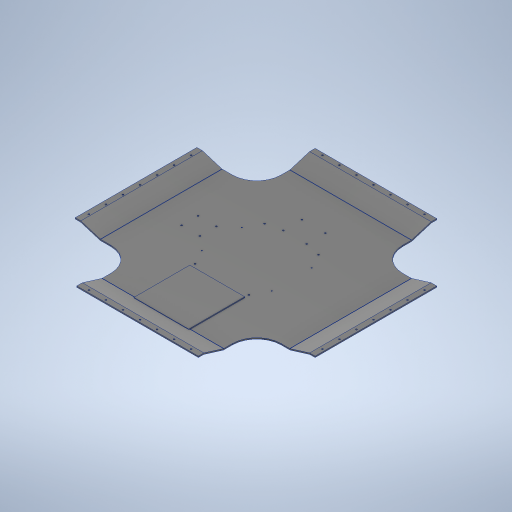
# Autodesk Inventor part: Swerve-Electronic-Plate
Saved by Autodesk Inventor 2024.2 (Build 282272000, 272)
## iProperties
Created: 2024-01-04
Part Number: Swerve-Electronic-Plate
Material: Aluminum 6061
Document SubType Name: Modeling
Designer: rohan
Density: 2.7 g/cm^3
Appearance: Aluminum - Flat
Author: rohan
Autodesk Inventor part; units mm, degrees
ref_plane "YZ Plane" through (0, 0, 0) normal (1, 0, 0) x (0, 1, 0)
ref_plane "XZ Plane" through (0, 0, 0) normal (0, 1, 0) x (-1, 0, 0)
ref_plane "XY Plane" through (0, 0, 0) normal (0, 0, 1) x (1, 0, 0)
sketch "Sketch6" plane through (0, 0, 0) normal (0, 1, 0) x (-1, 0, 0)
  line L0 (311.15, 311.15) -> (-311.15, 311.15)
  line L1 (-311.15, 311.15) -> (-311.15, -311.15)
  line L2 (-311.15, -311.15) -> (311.15, -311.15)
  line L3 (311.15, -311.15) -> (311.15, 311.15)
  line L4 (311.15, 311.15) -> (-311.15, -311.15) construction
  line L5 (-311.15, 311.15) -> (311.15, -311.15) construction
  point P0 (0, 0)
  dimension "d60" = 622.3
  dimension "d61" = 622.3
  constraints: 12 end point, 2 midpoint, 2 parallel, 1 horizontal, 1 perpendicular
  measures "d60" distance of L2.end L1.end
  measures "d61" distance of L1.end L0.end
extrude "Extrusion5" add sketch "Sketch6" along normal blind 3.175
sketch "Sketch7" plane through (0, 3.175, 0) normal (0, 1, 0) x (1, 0, 0)
  line L0 (311.15, -311.15) -> (311.15, 311.15) projected
  line L1 (311.15, 311.15) -> (-311.15, 311.15) projected
  line L2 (-311.15, 311.15) -> (-311.15, -311.15) projected
  line L3 (-311.15, -311.15) -> (311.15, -311.15) projected
  line L4 (-298.45, -298.45) -> (-298.45, 298.45)
  line L5 (-298.45, 298.45) -> (298.45, 298.45)
  line L6 (298.45, 298.45) -> (298.45, -298.45)
  line L7 (298.45, -298.45) -> (-298.45, -298.45)
  line L8 (0, -298.45) -> (0, -311.15)
  circle A0 centre (0, -304.8) radius 1.9939
  circle A1 centre (44.45, -304.8) radius 1.9939
  circle A2 centre (88.9, -304.8) radius 1.9939
  circle A3 centre (133.35, -304.8) radius 1.9939
  circle A4 centre (-44.45, -304.8) radius 1.9939
  circle A5 centre (0, -304.8) radius 1.9939
  circle A6 centre (44.45, -304.8) radius 1.9939
  circle A7 centre (88.9, -304.8) radius 1.9939
  circle A8 centre (-88.9, -304.8) radius 1.9939
  circle A9 centre (-44.45, -304.8) radius 1.9939
  circle A10 centre (0, -304.8) radius 1.9939
  circle A11 centre (44.45, -304.8) radius 1.9939
  circle A12 centre (-133.35, -304.8) radius 1.9939
  circle A13 centre (-88.9, -304.8) radius 1.9939
  circle A14 centre (-44.45, -304.8) radius 1.9939
  circle A15 centre (0, -304.8) radius 1.9939
  line L9 (-413.2249, 0) -> (395.3055, 0)
  line L10 (298.45, 298.45) -> (-298.45, 298.45)
  line L11 (0, 298.45) -> (0, 311.15)
  circle A16 centre (0, 304.8) radius 1.9939
  circle A17 centre (44.45, 304.8) radius 1.9939
  circle A18 centre (88.9, 304.8) radius 1.9939
  circle A19 centre (133.35, 304.8) radius 1.9939
  circle A20 centre (-44.45, 304.8) radius 1.9939
  circle A21 centre (0, 304.8) radius 1.9939
  circle A22 centre (44.45, 304.8) radius 1.9939
  circle A23 centre (88.9, 304.8) radius 1.9939
  circle A24 centre (-88.9, 304.8) radius 1.9939
  circle A25 centre (-44.45, 304.8) radius 1.9939
  circle A26 centre (0, 304.8) radius 1.9939
  circle A27 centre (44.45, 304.8) radius 1.9939
  circle A28 centre (-133.35, 304.8) radius 1.9939
  circle A29 centre (-88.9, 304.8) radius 1.9939
  circle A30 centre (-44.45, 304.8) radius 1.9939
  circle A31 centre (0, 304.8) radius 1.9939
  line L12 (-311.15, 0) -> (-298.45, 0)
  circle A32 centre (-304.8, 0) radius 1.9939
  circle A33 centre (-304.8, -44.45) radius 1.9939
  circle A34 centre (-304.8, -88.9) radius 1.9939
  circle A35 centre (-304.8, -133.35) radius 1.9939
  circle A36 centre (-304.8, 44.45) radius 1.9939
  circle A37 centre (-304.8, 0) radius 1.9939
  circle A38 centre (-304.8, -44.45) radius 1.9939
  circle A39 centre (-304.8, -88.9) radius 1.9939
  circle A40 centre (-304.8, 88.9) radius 1.9939
  circle A41 centre (-304.8, 44.45) radius 1.9939
  circle A42 centre (-304.8, 0) radius 1.9939
  circle A43 centre (-304.8, -44.45) radius 1.9939
  circle A44 centre (-304.8, 133.35) radius 1.9939
  circle A45 centre (-304.8, 88.9) radius 1.9939
  circle A46 centre (-304.8, 44.45) radius 1.9939
  circle A47 centre (-304.8, 0) radius 1.9939
  line L13 (0, 372.2506) -> (0, -355.6631)
  circle A48 centre (304.8, 0) radius 1.9939
  circle A49 centre (304.8, -44.45) radius 1.9939
  circle A50 centre (304.8, -88.9) radius 1.9939
  circle A51 centre (304.8, -133.35) radius 1.9939
  circle A52 centre (304.8, 44.45) radius 1.9939
  circle A53 centre (304.8, 0) radius 1.9939
  circle A54 centre (304.8, -44.45) radius 1.9939
  circle A55 centre (304.8, -88.9) radius 1.9939
  circle A56 centre (304.8, 88.9) radius 1.9939
  circle A57 centre (304.8, 44.45) radius 1.9939
  circle A58 centre (304.8, 0) radius 1.9939
  circle A59 centre (304.8, -44.45) radius 1.9939
  circle A60 centre (304.8, 133.35) radius 1.9939
  circle A61 centre (304.8, 88.9) radius 1.9939
  circle A62 centre (304.8, 44.45) radius 1.9939
  circle A63 centre (304.8, 0) radius 1.9939
  point P0 (0, 0)
  dimension "d64" = 12.7
  dimension "d65" = 3.9878
  dimension "d68" = 44.45
  dimension "d71" = 44.45
  dimension "d74" = 3.9878
  dimension "d77" = 44.45
  dimension "d80" = 44.45
  constraints: 64 centre point, 34 symmetric about line, 20 end point, 6 midpoint, 3 horizontal, 2 point on line, 2 vertical, 1 perpendicular, 95 other
  measures "d64" distance between parallel lines of L2 L4
  measures "d65" diameter of A0
  measures "d68" distance of A0.centre A1.centre
  measures "d71" distance of A0.centre A4.centre
  measures "d74" diameter of A32
  measures "d77" distance of A32.centre A33.centre
  measures "d80" distance of A32.centre A36.centre
extrude "Extrusion6" cut sketch "Sketch7" against normal blind 3.175 contours A48 L9 | L9 A48 | A0 L8 | L8 A0 | A16 L11 | L11 A16 | A32 L9 | L9 A32 | A1 | A2 | A3 | A4 | A8 | A12 | A17 | A18 | A19 | A20 | A24 | A28 | A33 | A34 | A35 | A36 | A40 | A44 | A49 | A50 | A51 | A52 | A56 | A60
sketch "Sketch8" plane through (0, 3.175, 0) normal (0, 1, 0) x (1, 0, 0)
  line L0 (-311.15, 311.15) -> (-311.15, -311.15) projected
  circle A0 centre (-304.8, 88.9) radius 1.9939 projected
  circle A1 centre (-304.8, -133.35) radius 1.9939 projected
  circle A2 centre (0, -304.8) radius 1.9939 projected
  circle A3 centre (304.8, -133.35) radius 1.9939 projected
  circle A4 centre (304.8, 44.45) radius 1.9939 projected
  circle A5 centre (88.9, 304.8) radius 1.9939 projected
  circle A6 centre (-88.9, 304.8) radius 1.9939 projected
  circle A7 centre (-44.45, 304.8) radius 1.9939 projected
  circle A8 centre (133.35, 304.8) radius 1.9939 projected
  circle A9 centre (304.8, 0) radius 1.9939 projected
  circle A10 centre (133.35, -304.8) radius 1.9939 projected
  circle A11 centre (-44.45, -304.8) radius 1.9939 projected
  circle A12 centre (-304.8, -88.9) radius 1.9939 projected
  circle A13 centre (-304.8, 133.35) radius 1.9939 projected
  circle A14 centre (-304.8, 44.45) radius 1.9939 projected
  circle A15 centre (-133.35, -304.8) radius 1.9939 projected
  circle A16 centre (44.45, -304.8) radius 1.9939 projected
  circle A17 centre (304.8, -88.9) radius 1.9939 projected
  circle A18 centre (304.8, 88.9) radius 1.9939 projected
  circle A19 centre (44.45, 304.8) radius 1.9939 projected
  circle A20 centre (-133.35, 304.8) radius 1.9939 projected
  circle A21 centre (0, 304.8) radius 1.9939 projected
  circle A22 centre (304.8, 133.35) radius 1.9939 projected
  circle A23 centre (304.8, -44.45) radius 1.9939 projected
  circle A24 centre (88.9, -304.8) radius 1.9939 projected
  circle A25 centre (-88.9, -304.8) radius 1.9939 projected
  circle A26 centre (-304.8, -44.45) radius 1.9939 projected
  circle A27 centre (-304.8, 0) radius 1.9939 projected
  line L1 (311.15, -311.15) -> (311.15, 311.15) projected
  line L2 (311.15, 311.15) -> (-311.15, 311.15) projected
  line L3 (-311.15, 311.15) -> (-311.15, -311.15) projected
  line L4 (-311.15, -311.15) -> (311.15, -311.15) projected
  line L5 (311.15, 311.15) -> (-311.15, 311.15) projected
  line L6 (-158.75, 311.15) -> (-158.75, 222.25)
  line L7 (-222.25, 158.75) -> (-311.15, 158.75)
  line L8 (-311.15, -158.75) -> (-222.25, -158.75)
  line L9 (-158.75, -222.25) -> (-158.75, -311.15)
  line L10 (158.75, 311.15) -> (158.75, 222.25)
  line L11 (222.25, 158.75) -> (311.15, 158.75)
  line L12 (158.75, -311.15) -> (158.75, -222.25)
  line L13 (222.25, -158.75) -> (311.15, -158.75)
  arc A28 (-222.25, 158.75) -> (-158.75, 222.25) centre (-222.25, 222.25) ccw
  arc A29 (158.75, 222.25) -> (222.25, 158.75) centre (222.25, 222.25) ccw
  arc A30 (222.25, -158.75) -> (158.75, -222.25) centre (222.25, -222.25) ccw
  arc A31 (-158.75, -222.25) -> (-222.25, -158.75) centre (-222.25, -222.25) ccw
  point P0 (0, 0)
  point P1 (-311.15, 0)
  point P2 (0, 311.15)
  point P3 (-158.75, 158.75)
  point P4 (-158.75, -158.75)
  point P5 (158.75, 158.75)
  point P6 (0, -311.15)
  point P7 (158.75, -158.75)
  dimension "d93" = 63.5
  constraints: 18 point on line, 16 end point, 8 point on circle, 8 tangent, 4 centre point, 3 equal radius, 3 midpoint, 2 parallel, 2 perpendicular, 2 vertical
  measures "d93" radius of A28
extrude "Extrusion8" cut sketch "Sketch8" against normal blind 61.9125 contours L2 L6 A28 L7 L0 | L8 A31 L9 L4 L0 | L2 L1 L11 A29 L10 | L12 A30 L13 L1 L4
sketch "Sketch17" plane through (158.75, 3.175, 311.15) normal (1, 0, 0) x (0, 0, -1)
  line L0 (88.9, -3.175) -> (0, -3.175) projected
  line L1 (88.9, -3.175) -> (0, -3.175) projected
  line L2 (88.9, 0) -> (88.9, -3.175) projected
  line L3 (0, 0) -> (88.9, 0) projected
  line L4 (0, -3.175) -> (0, 0) projected
  line L5 (622.3, -3.175) -> (533.4, -3.175) projected
  line L6 (622.3, 0) -> (622.3, -3.175) projected
  line L7 (533.4, 0) -> (622.3, 0) projected
  line L8 (533.4, 0) -> (533.4, -3.175) projected
  line L9 (4.3561, 0) -> (8.3439, 0) projected
  line L10 (0, 12.7) -> (13.97, 12.7)
  line L11 (13.97, 12.7) -> (55.1332, 0)
  line L12 (152.4, 0) -> (469.9, 0) projected
  line L13 (311.15, 0) -> (311.15, 175.4287)
  line L14 (622.3, 12.7) -> (608.33, 12.7)
  line L15 (608.33, 12.7) -> (567.1668, 0)
  line L16 (56.0693, 3.0339) -> (14.4487, 15.875)
  line L17 (14.4487, 15.875) -> (0, 15.875)
  line L18 (51.3204, 4.499) -> (65.9027, 0)
  line L19 (0, 12.7) -> (0, 15.875)
  line L20 (622.3, 12.7) -> (608.33, 12.7)
  line L21 (608.33, 12.7) -> (567.1668, 0)
  line L22 (566.2307, 3.0339) -> (607.8513, 15.875)
  line L23 (607.8513, 15.875) -> (622.3, 15.875)
  line L24 (570.9796, 4.499) -> (556.3973, 0)
  line L25 (622.3, 12.7) -> (622.3, 15.875)
  point P0 (311.15, -3.175)
  point P1 (567.1668, 0)
  point P2 (56.0693, 3.0339)
  dimension "d150" = 13.97
  dimension "d151" = 13.97
  dimension "d152" = 3.175
  dimension "d153" = 12.7
  constraints: 30 end point, 8 symmetric about line, 6 point on line, 1 midpoint, 1 perpendicular, 1 vertical
  measures "d150" distance of L10.start L10.end
  measures "d151" distance of L14.start L15.start
  measures "d152" distance between parallel lines of L11 L16
  measures "d153" distance of L3.start L10.start
extrude "Extrusion17" add sketch "Sketch17" against normal up to surface (317.5 mm away) contours L3 L11 L10 L19 L17 L16 L18 | L7 L24 L22 L23 L25 L14 L15
sketch "Sketch18" plane through (311.15, 3.175, -158.75) normal (0, 0, -1) x (-1, 0, 0)
  line L0 (88.9, -3.175) -> (0, -3.175) projected
  line L1 (88.9, 0) -> (88.9, -3.175) projected
  line L2 (0, 0) -> (88.9, 0) projected
  line L3 (0, -3.175) -> (0, 0) projected
  line L4 (622.3, -3.175) -> (533.4, -3.175) projected
  line L5 (622.3, 0) -> (622.3, -3.175) projected
  line L6 (533.4, 0) -> (622.3, 0) projected
  line L7 (533.4, 0) -> (533.4, -3.175) projected
  line L8 (152.4, 0) -> (469.9, 0) projected
  line L9 (309.1561, 0) -> (313.1439, 0) projected
  line L10 (313.1439, 0) -> (313.1439, 161.3413)
  line L11 (0, 12.7) -> (13.97, 12.7)
  line L12 (13.97, 12.7) -> (55.1338, 0)
  line L13 (88.9, 0) -> (0, 0) projected
  line L14 (56.0698, 3.0339) -> (14.4486, 15.875)
  line L15 (14.4486, 15.875) -> (0, 15.875)
  line L16 (0, 12.7) -> (0, 15.875)
  line L17 (54.6659, 3.467) -> (65.9034, 0)
  line L18 (626.2878, 12.7) -> (612.3178, 12.7)
  line L19 (612.3178, 12.7) -> (571.154, 0)
  line L20 (570.218, 3.0339) -> (611.8392, 15.875)
  line L21 (611.8392, 15.875) -> (626.2878, 15.875)
  line L22 (626.2878, 12.7) -> (626.2878, 15.875)
  line L23 (571.6219, 3.467) -> (560.3844, 0)
  point P0 (311.15, -3.175)
  point P1 (571.154, 0)
  point P2 (55.1338, 0)
  point P3 (56.0698, 3.0339)
  dimension "d157" = 13.97
  dimension "d158" = 43.0784
  dimension "d159" = 3.175
  dimension "d160" = 12.7
  constraints: 26 end point, 8 symmetric about line, 6 point on line, 1 perpendicular, 1 vertical
  measures "d157" distance of L11.start L11.end
  measures "d158" distance of L11.end L12.end
  measures "d159" distance between parallel lines of L12 L14
  measures "d160" distance of L11.start L2.start
extrude "Extrusion18" add sketch "Sketch18" against normal up to surface (317.5 mm away) contours L2 L12 L11 L16 L15 L14 L17 | L6 L23 L20 L21 L22 L18 L19
sketch "Sketch19" plane through (296.7014, 19.05, -158.75) normal (0, 1, 0) x (1, 0, 0)
  line L0 (-455.4514, -469.9) -> (-455.4514, -455.4513) projected
  line L1 (-137.9514, -469.9) -> (-455.4514, -469.9) projected
  line L2 (-137.9514, -455.4513) -> (-137.9514, -469.9) projected
  line L3 (-137.9514, -455.4513) -> (-455.4514, -455.4513) projected
  line L4 (14.4486, -317.5) -> (0, -317.5) projected
  line L5 (14.4486, 0) -> (14.4486, -317.5) projected
  line L6 (0, 0) -> (14.4486, 0) projected
  line L7 (0, 0) -> (0, -317.5) projected
  line L8 (-597.3905, -317.5) -> (-611.8392, -317.5) projected
  line L9 (-597.3905, 0) -> (-597.3905, -317.5) projected
  line L10 (-611.8392, 0) -> (-597.3905, 0) projected
  line L11 (-611.8392, 0) -> (-611.8392, -317.5) projected
  line L12 (-455.4514, 137.9513) -> (-455.4514, 152.4) projected
  line L13 (-137.9514, 137.9513) -> (-455.4514, 137.9513) projected
  line L14 (-137.9514, 152.4) -> (-137.9514, 137.9513) projected
  line L15 (-137.9514, 152.4) -> (-455.4514, 152.4) projected
  circle A0 centre (-163.3514, -463.55) radius 1.9939 projected
  circle A1 centre (-207.8014, -463.55) radius 1.9939 projected
  circle A2 centre (-252.2514, -463.55) radius 1.9939 projected
  circle A3 centre (-296.7014, -463.55) radius 1.9939 projected
  circle A4 centre (-341.1514, -463.55) radius 1.9939 projected
  circle A5 centre (-385.6014, -463.55) radius 1.9939 projected
  circle A6 centre (-430.0514, -463.55) radius 1.9939 projected
  circle A7 centre (8.0986, -292.1) radius 1.9939 projected
  circle A8 centre (8.0986, -247.65) radius 1.9939 projected
  circle A9 centre (8.0986, -203.2) radius 1.9939 projected
  circle A10 centre (8.0986, -158.75) radius 1.9939 projected
  circle A11 centre (8.0986, -114.3) radius 1.9939 projected
  circle A12 centre (8.0986, -69.85) radius 1.9939 projected
  circle A13 centre (8.0986, -25.4) radius 1.9939 projected
  line L16 (-611.8392, -158.75) -> (14.4486, -158.75)
  line L17 (-296.7014, -469.9) -> (-296.7014, 152.4)
  circle A14 centre (-163.3514, 146.05) radius 1.9939
  circle A15 centre (-207.8014, 146.05) radius 1.9939
  circle A16 centre (-252.2514, 146.05) radius 1.9939
  circle A17 centre (-296.7014, 146.05) radius 1.9939
  circle A18 centre (-341.1514, 146.05) radius 1.9939
  circle A19 centre (-385.6014, 146.05) radius 1.9939
  circle A20 centre (-430.0514, 146.05) radius 1.9939
  circle A21 centre (-601.5014, -292.1) radius 1.9939
  circle A22 centre (-601.5014, -247.65) radius 1.9939
  circle A23 centre (-601.5014, -203.2) radius 1.9939
  circle A24 centre (-601.5014, -158.75) radius 1.9939
  circle A25 centre (-601.5014, -114.3) radius 1.9939
  circle A26 centre (-601.5014, -69.85) radius 1.9939
  circle A27 centre (-601.5014, -25.4) radius 1.9939
  point P0 (-296.7014, -158.75)
  constraints: 14 centre point, 14 symmetric about line, 4 end point, 4 midpoint, 14 other
sketch "Sketch20" plane through (158.75, 0, 222.25) normal (1, 0, 0) x (0, 0, -1)
  line L0 (-88.9, 3.175) -> (-33.7668, 3.175) projected
  line L1 (-88.9, 0) -> (-88.9, 3.175) projected
  line L2 (0, 0) -> (-88.9, 0) projected
  line L3 (478.2668, 3.175) -> (533.4, 3.175) projected
  line L4 (533.4, 3.175) -> (533.4, 0) projected
  line L5 (533.4, 0) -> (444.5, 0) projected
  line L6 (478.2668, 3.175) -> (519.43, 15.875) projected
  line L7 (501.2942, 10.2796) -> (461.0855, -2.1259)
  line L8 (-74.93, 15.875) -> (-33.7668, 3.175) projected
  line L9 (-50.6777, 8.3925) -> (-16.5855, -2.1259)
  point P0 (222.25, 0)
  point P1 (467.9759, 0)
  point P2 (-23.4759, 0)
  constraints: 4 end point, 4 point on line
extrude "Extrusion19" cut sketch "Sketch20" against normal up to surface (317.5 mm away)
sketch "Sketch21" plane through (222.25, 0, 158.75) normal (0, 0, 1) x (1, 0, 0)
  line L0 (-523.4178, 15.875) -> (-482.254, 3.175) projected
  line L1 (-533.4, 3.175) -> (-482.254, 3.175) projected
  line L2 (-533.4, 0) -> (-533.4, 3.175) projected
  line L3 (-444.5, 0) -> (-533.4, 0) projected
  line L4 (33.7662, 3.175) -> (74.93, 15.875) projected
  line L5 (33.7662, 3.175) -> (88.9, 3.175) projected
  line L6 (88.9, 3.175) -> (88.9, 0) projected
  line L7 (88.9, 0) -> (0, 0) projected
  line L8 (58.6751, 10.86) -> (20.8324, -0.8154)
  line L9 (-502.8359, 9.525) -> (-462.2068, -3.01)
  point P0 (-222.25, 0)
  point P1 (-471.963, 0)
  point P2 (23.4752, 0)
  constraints: 4 end point, 2 point on line, 1 midpoint
extrude "Extrusion20" cut sketch "Sketch21" against normal blind 396.875
extrude "Extrusion21" cut sketch "Sketch19" against normal blind 111.125 contours L17 A3 | A3 L17 | L16 A10 | A10 L16 | A24 L16 | L16 A24 | A17 L17 | L17 A17 | A0 | A1 | A2 | A4 | A5 | A6 | A7 | A8 | A9 | A11 | A12 | A13 | A14 | A15 | A16 | A18 | A19 | A20 | A21 | A22 | A23 | A25 | A26 | A27
fillet "Fillet1" radius 3.175 4 edges at (0, 3.175, 245.2473) (245.2466, 3.175, 0) (0, 3.175, -245.2473) (-249.2344, 3.175, 0)
sketch "Sketch24" plane through (0, 3.175, 0) normal (0, 1, 0) x (1, 0, 0)
  line L0 (70.2691, -90.8431) -> (-70.2691, -90.8431)
  line L1 (-70.2691, -90.8431) -> (-70.2691, 90.8431)
  line L2 (-70.2691, 90.8431) -> (70.2691, 90.8431)
  line L3 (70.2691, 90.8431) -> (70.2691, -90.8431)
  line L4 (70.2691, -90.8431) -> (-70.2691, 90.8431) construction
  line L5 (-70.2691, -90.8431) -> (70.2691, 90.8431) construction
  circle A0 centre (-70.2691, -90.8431) radius 1.9939
  circle A1 centre (70.2691, -90.8431) radius 1.9939
  circle A2 centre (70.2691, 90.8431) radius 1.9939
  circle A3 centre (-70.2691, 90.8431) radius 1.9939
  point P0 (0, 0)
  dimension "d174" = 140.5382
  dimension "d175" = 181.6862
  dimension "d176" = 3.9878
  dimension "d177" = 3.9878
  dimension "d178" = 3.9878
  dimension "d179" = 3.9878
  constraints: 12 end point, 4 centre point, 4 coincident, 2 midpoint, 2 parallel, 1 horizontal, 1 perpendicular
  measures "d174" distance of L1.end L2.end
  measures "d175" distance of L0.end L1.end
  measures "d176" diameter of A0
  measures "d177" diameter of A1
  measures "d178" diameter of A2
  measures "d179" diameter of A3
extrude "Extrusion24" cut sketch "Sketch24" against normal blind 30.1625 contours A0 L1 L0 | L0 L1 A0 | A1 L3 L0 | L0 L3 A1 | A3 L2 L1 | L1 L2 A3 | A2 L2 L3 | L3 L2 A2
sketch "Sketch26" plane through (0, 3.175, 0) normal (0, 1, 0) x (1, 0, 0)
  line L0 (91.1352, -52.197) -> (-91.1352, -52.197)
  line L1 (-91.1352, -52.197) -> (-91.1352, 52.197)
  line L2 (-91.1352, 52.197) -> (91.1352, 52.197)
  line L3 (91.1352, 52.197) -> (91.1352, -52.197)
  line L4 (91.1352, -52.197) -> (-91.1352, 52.197) construction
  line L5 (-91.1352, -52.197) -> (91.1352, 52.197) construction
  circle A0 centre (-91.1352, -52.197) radius 1.3462
  circle A1 centre (-91.1352, 52.197) radius 1.3462
  circle A2 centre (91.1352, -52.197) radius 1.3462
  circle A3 centre (91.1352, 52.197) radius 1.3462
  point P0 (0, 0)
  dimension "d74" = 3.9878
  dimension "d184" = 182.2704
  dimension "d185" = 104.394
  dimension "d186" = 2.6924
  dimension "d187" = 2.6924
  dimension "d188" = 2.6924
  constraints: 12 end point, 4 centre point, 4 coincident, 2 midpoint, 2 parallel, 1 horizontal, 1 perpendicular
  measures "d184" distance of L1.end L2.end
  measures "d185" distance of L0.end L1.end
  measures "d186" diameter of A0
  measures "d187" diameter of A1
  measures "d188" diameter of A2
extrude "Extrusion26" cut sketch "Sketch26" against normal blind 15.875 contours A0 L1 L0 | L0 L1 A0 | A2 L3 L0 | L0 L3 A2 | A1 L2 L1 | L1 L2 A1 | A3 L2 L3 | L3 L2 A3
sketch "Sketch27" plane through (0, 3.175, 0) normal (0, 1, 0) x (1, 0, 0)
  line L0 (0, 0) -> (0, 124.0934)
  line L1 (30.5181, 99.6713) -> (-30.5181, 99.6713)
  line L2 (-30.5181, 99.6713) -> (-30.5181, 148.5155)
  line L3 (-30.5181, 148.5155) -> (30.5181, 148.5155)
  line L4 (30.5181, 148.5155) -> (30.5181, 99.6713)
  line L5 (30.5181, 99.6713) -> (-30.5181, 148.5155) construction
  line L6 (-30.5181, 99.6713) -> (30.5181, 148.5155) construction
  circle A0 centre (-30.5181, 99.6713) radius 1.8923
  circle A1 centre (-30.5181, 148.5155) radius 1.8923
  circle A2 centre (30.5181, 148.5155) radius 1.8923
  circle A3 centre (30.5181, 99.6713) radius 1.8923
  dimension "d191" = 61.0362
  dimension "d192" = 48.8442
  dimension "d193" = 3.7846
  dimension "d194" = 3.7846
  constraints: 14 end point, 4 centre point, 4 coincident, 2 midpoint, 2 parallel, 1 horizontal, 1 perpendicular, 1 vertical
  measures "d191" distance of L2.end L3.end
  measures "d192" distance of L1.end L2.end
  measures "d193" diameter of A0
  measures "d194" diameter of A1
extrude "Extrusion27" cut sketch "Sketch27" against normal blind 42.8625 contours A0 L2 L1 | L1 L2 A0 | A3 L4 L1 | L1 L4 A3 | A1 L3 L2 | L2 L3 A1 | A2 L3 L4 | L4 L3 A2
sketch "Sketch28" plane through (0, 3.175, 0) normal (0, 1, 0) x (1, 0, 0)
  line L0 (0, 0) -> (-150.791, 0)
  line L1 (-174.667, -21.5265) -> (-126.915, -21.5265)
  line L2 (-126.915, -21.5265) -> (-126.915, 21.5265)
  line L3 (-126.915, 21.5265) -> (-174.667, 21.5265)
  line L4 (-174.667, 21.5265) -> (-174.667, -21.5265)
  line L5 (-174.667, -21.5265) -> (-126.915, 21.5265) construction
  line L6 (-126.915, -21.5265) -> (-174.667, 21.5265) construction
  circle A0 centre (-174.667, -21.5265) radius 1.9939
  circle A1 centre (-174.667, 21.5265) radius 1.9939
  circle A2 centre (-126.915, -21.5265) radius 1.9939
  circle A3 centre (-126.915, 21.5265) radius 1.9939
  dimension "d197" = 47.752
  dimension "d198" = 43.053
  dimension "d199" = 3.9878
  dimension "d200" = 3.9878
  dimension "d201" = 3.9878
  dimension "d202" = 3.9878
  constraints: 14 end point, 4 centre point, 4 coincident, 2 horizontal, 2 midpoint, 2 parallel, 1 perpendicular
  measures "d197" distance of L3.end L2.end
  measures "d198" distance of L3.end L1.start
  measures "d199" diameter of A0
  measures "d200" diameter of A1
  measures "d201" diameter of A2
  measures "d202" diameter of A3
extrude "Extrusion28" cut sketch "Sketch28" against normal blind 11.1125 contours L4 A0 L1 | L1 A0 L4 | A2 L2 L1 | L1 L2 A2 | A1 L3 L4 | L4 L3 A1 | A3 L2 L3 | L3 L2 A3
sketch "Sketch29" plane through (0, 3.175, 0) normal (0, 1, 0) x (1, 0, 0)
  line L0 (71.5899, -103.1082) -> (-71.5899, -103.1082)
  line L1 (-71.5899, -103.1082) -> (-71.5899, -249.2598)
  line L2 (-71.5899, -249.2598) -> (71.5899, -249.2598)
  line L3 (71.5899, -249.2598) -> (71.5899, -103.1082)
  line L4 (71.5899, -103.1082) -> (-71.5899, -249.2598) construction
  line L5 (-71.5899, -103.1082) -> (71.5899, -249.2598) construction
  point P0 (0, 0)
  point P1 (0, -176.184)
  dimension "d205" = 143.1798
  dimension "d206" = 146.1516
  constraints: 12 end point, 2 midpoint, 2 parallel, 1 horizontal, 1 perpendicular
  measures "d205" distance of L2.end L1.end
  measures "d206" distance of L1.end L0.end
extrude "Extrusion29" add sketch "Sketch29" along normal blind 2.54
body "Solid2"
